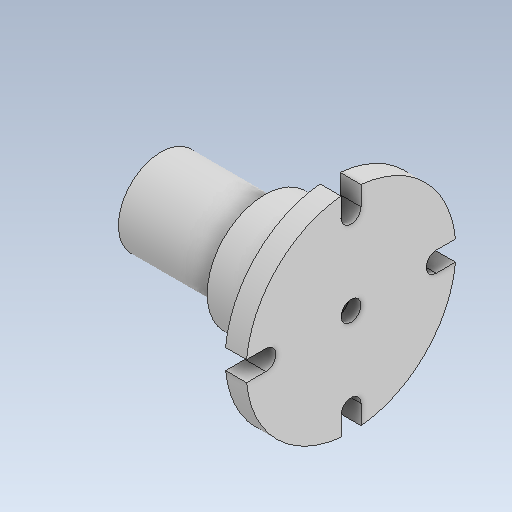
# Autodesk Inventor part: wheel_adapter_inner
Saved by Autodesk Inventor 2021 (Build 250183000, 183)
## iProperties
Created: 2020-12-08
Part Number: wheel_adapter_inner
Material: Generic
Document SubType Name: Modeling
Designer: Mateusz
Density: 1 g/cm^3
Appearance: Default
Author: Mateusz
Autodesk Inventor part; units mm, degrees
ref_plane "YZ Plane" through (0, 0, 0) normal (1, 0, 0) x (0, 1, 0)
ref_plane "XZ Plane" through (0, 0, 0) normal (0, 1, 0) x (-1, 0, 0)
sketch "Sketch1" plane through (0, 0, 0) normal (1, 0, 0) x (0, 1, 0)
  circle A0 centre (0, 0) radius 19.25
  circle A1 centre (0, 0) radius 17.25
  circle A2 centre (0, 0) radius 22.25
  dimension "d0" = 38.5
  dimension "d1" = 34.5
  dimension "d6" = 44.5
  constraints: 3 centre point, 3 coincident
  measures "d0" diameter of A0
  measures "d1" diameter of A1
  measures "d6" diameter of A2
extrude "Extrusion1" add sketch "Sketch1" along normal blind 5 contours A0 | A1 | A2
extrude "Extrusion2" add sketch "Sketch1" against normal blind 71 contours A1
extrude "Extrusion3" add sketch "Sketch1" against normal blind 34 contours A2
sketch "Sketch2" plane through (5, 0, 0) normal (1, 0, 0) x (0, 0, -1)
  line L0 (0, -7.5) -> (-6.4952, -3.75)
  line L1 (-6.4952, -3.75) -> (-6.4952, 3.75)
  line L2 (-6.4952, 3.75) -> (0, 7.5)
  line L3 (0, 7.5) -> (6.4952, 3.75)
  line L4 (6.4952, 3.75) -> (6.4952, -3.75)
  line L5 (6.4952, -3.75) -> (0, -7.5)
  constraints: 12 end point
extrude "Extrusion4" cut sketch "Sketch2" against normal through all
sketch "Sketch3" plane through (-34, 0, 0) normal (-1, 0, 0) x (0, 0, 1)
  circle A0 centre (0, 0) radius 42.5
  circle A1 centre (0, 0) radius 22.25 projected
  dimension "d12" = 85
  constraints: 1 centre point, 1 coincident
  measures "d12" diameter of A0
extrude "Extrusion5" add sketch "Sketch3" against normal blind 5
sketch "Sketch4" plane through (5, 0, 0) normal (1, 0, 0) x (0, 0, -1)
  line L0 (0, -7.5) -> (-6.4952, -3.75) projected
  line L1 (-6.4952, -3.75) -> (-6.4952, 3.75) projected
  line L2 (-6.4952, 3.75) -> (0, 7.5) projected
  line L3 (0, 7.5) -> (6.4952, 3.75) projected
  line L4 (6.4952, 3.75) -> (6.4952, -3.75) projected
  line L5 (6.4952, -3.75) -> (0, -7.5) projected
  circle A0 centre (0, 0) radius 4.05
  dimension "d15" = 8.1
  constraints: 1 centre point, 1 coincident
  measures "d15" diameter of A0
extrude "Extrusion6" add sketch "Sketch4" against normal blind 4
ref_plane "Work Plane1" through (-29, 0, 0) normal (1, 0, 0) x (0, 0, -1)
sketch "Sketch5" plane through (-29, 0, 0) normal (1, 0, 0) x (0, 0, -1)
  line L0 (0, 0) -> (34.5, 0)
  circle A0 centre (34.5, 0) radius 4.05
  circle A1 centre (0, 34.5) radius 4.05
  circle A2 centre (-34.5, 0) radius 4.05
  circle A3 centre (0, -34.5) radius 4.05
  dimension "d19" = 34.5
  dimension "d20" = 8.1
  dimension "d23" = 360
  constraints: 4 centre point, 2 end point, 1 coincident, 1 horizontal, 9 other
  measures "d19" distance of L0.start L0.end
  measures "d20" diameter of A0
extrude "Extrusion7" cut sketch "Sketch5" against normal up to surface (5 mm away)
sketch "Sketch6" plane through (5, 0, 0) normal (1, 0, 0) x (0, 0, -1)
  circle A0 centre (0, 0) radius 22.25 projected
  circle A1 centre (0, 0) radius 23.25
  dimension "d27" = 46.5
  constraints: 1 centre point, 1 coincident
  measures "d27" diameter of A1
extrude "Extrusion8" add sketch "Sketch6" against normal up to surface (34 mm away)
sketch "Sketch7" plane through (5, 0, 0) normal (1, 0, 0) x (0, 0, -1)
  circle A0 centre (0, 0) radius 23.25 projected
  circle A1 centre (0, -34.5) radius 4.05 projected
  circle A2 centre (0, 34.5) radius 4.05 projected
  circle A3 centre (34.5, 0) radius 4.05 projected
  circle A4 centre (-34.5, 0) radius 4.05 projected
  circle A5 centre (0, 0) radius 42.5 projected
extrude "Extrusion9" add sketch "Sketch7" against normal blind 5
sketch "Sketch8" plane through (-34, 0, 0) normal (-1, 0, 0) x (0, 0, 1)
  circle A0 centre (0, -34.5) radius 4.05 projected
  circle A1 centre (0, 34.5) radius 4.05 projected
  circle A2 centre (-34.5, 0) radius 4.05 projected
  circle A3 centre (34.5, 0) radius 4.05 projected
  circle A4 centre (0, 0) radius 42.5 projected
  circle A5 centre (0, 0) radius 19.25 projected
extrude "Extrusion10" cut sketch "Sketch8" against normal up to surface (5 mm away)
sketch "Sketch9" plane through (5, 0, 0) normal (1, 0, 0) x (0, 0, -1)
  circle A0 centre (0, -34.5) radius 4.05 projected
  circle A1 centre (0, 34.5) radius 4.05 projected
  circle A2 centre (34.5, 0) radius 4.05 projected
  circle A3 centre (-34.5, 0) radius 4.05 projected
  circle A4 centre (0, 0) radius 42.5 projected
  circle A5 centre (0, 0) radius 4.05 projected
extrude "Extrusion11" add sketch "Sketch9" along normal blind 1
sketch "Sketch10" plane through (0, 0, 0) normal (-1, 0, 0) x (0, 0, 1)
  circle A0 centre (0, 0) radius 42.5 projected
  circle A1 centre (34.5, 0) radius 4.05 projected
  circle A2 centre (-34.5, 0) radius 4.05 projected
  circle A3 centre (0, 34.5) radius 4.05 projected
  circle A4 centre (0, -34.5) radius 4.05 projected
  circle A5 centre (0, 0) radius 23.25 projected
extrude "Extrusion12" add sketch "Sketch10" along normal blind 2.5
sketch "Sketch11" plane through (6, 0, 0) normal (1, 0, 0) x (0, 0, -1)
  circle A0 centre (0, 34.5) radius 4.05 projected
  line L0 (-4.05, 34.5) -> (-4.05, 42.3066)
  line L1 (4.05, 34.5) -> (4.05, 42.3066)
  circle A1 centre (0, 0) radius 42.5 projected
  arc A2 (4.05, 34.5) -> (-4.05, 34.5) centre (0, 34.5) ccw
  circle A3 centre (0, 0) radius 4.05 projected
  arc A4 (4.05, 42.3066) -> (-4.05, 42.3066) centre (0, 0) ccw
  line L2 (-34.5, -4.05) -> (-42.3066, -4.05)
  line L3 (-34.5, 4.05) -> (-42.3066, 4.05)
  arc A5 (-34.5, 4.05) -> (-34.5, -4.05) centre (-34.5, 0) ccw
  arc A6 (-42.3066, 4.05) -> (-42.3066, -4.05) centre (0, 0) ccw
  line L4 (4.05, -34.5) -> (4.05, -42.3066)
  line L5 (-4.05, -34.5) -> (-4.05, -42.3066)
  arc A7 (-4.05, -34.5) -> (4.05, -34.5) centre (0, -34.5) ccw
  arc A8 (-4.05, -42.3066) -> (4.05, -42.3066) centre (0, 0) ccw
  line L6 (34.5, 4.05) -> (42.3066, 4.05)
  line L7 (34.5, -4.05) -> (42.3066, -4.05)
  arc A9 (34.5, -4.05) -> (34.5, 4.05) centre (34.5, 0) ccw
  arc A10 (42.3066, -4.05) -> (42.3066, 4.05) centre (0, 0) ccw
  dimension "d40" = 360
  constraints: 19 point on circle, 16 end point, 8 centre point, 5 coincident, 2 concentric, 2 vertical, 45 other
extrude "Extrusion13" cut sketch "Sketch11" against normal up to surface (8.5 mm away) contours A0 L0 A1 L1 | A1 L7 A9 L6 | L3 A5 L2 A1 | L5 A7 L4 A1
sketch "Sketch12" plane through (1, 0, 0) normal (-1, 0, 0) x (0, 0, 1)
  point P0 (0, 0)
body "Solid1"
